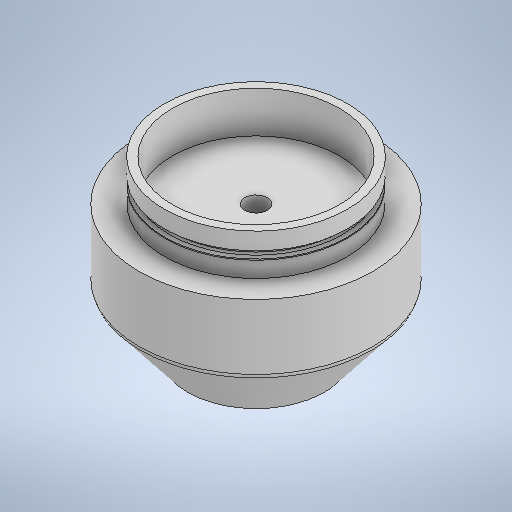
# Autodesk Inventor part: cap_v0.7.0
Saved by Autodesk Inventor 2025 (Build 290162000, 162)
## iProperties
Created: 2026-01-06
Part Number: cap_v0.7.0
Material: Generic
Document SubType Name: Modeling
Designer: SLM30
Density: 1 g/cm^3
Appearance: Default
Author: SLM30
Autodesk Inventor part; units mm, degrees
ref_plane "YZ Plane" through (0, 0, 0) normal (1, 0, 0) x (0, 1, 0)
ref_plane "XZ Plane" through (0, 0, 0) normal (0, 1, 0) x (-1, 0, 0)
ref_plane "XY Plane" through (0, 0, 0) normal (0, 0, 1) x (1, 0, 0)
sketch "Sketch1" plane through (0, 0, 0) normal (0, 0, 1) x (1, 0, 0)
  line L0 (0, 0) -> (-15, 0)
  line L1 (-15, 0) -> (-15, 11)
  line L2 (-15, 11) -> (-0.0863, 11)
  line L3 (-0.0863, 11) -> (-0.0863, 21)
  line L4 (-0.0863, 21) -> (-26.0863, 21)
  line L5 (-26.0863, 21) -> (-26.0863, 25.2964)
  line L6 (-26.0863, 25.2964) -> (-27.3219, 25.2964)
  line L7 (-28.5, 25.9476) -> (-28.5, 21)
  line L8 (-28.5, 21) -> (-36.5, 21)
  line L9 (-36.5, 21) -> (-36.5, 0)
  line L10 (-36.5, 0) -> (0, 0)
  line L11 (0, 0) -> (0, 0)
  line L12 (-36.5, 0) -> (-20.7775, -20)
  line L13 (-20.7775, -20) -> (0, -20)
  line L14 (0, -20) -> (0, 0)
  line L15 (-26.0863, 25.2964) -> (-26.0863, 33.8784)
  line L16 (-26.0863, 33.8784) -> (-28.5863, 33.8784)
  line L17 (-28.5863, 33.8784) -> (-28.5, 25.9476)
  arc A0 (-26.6145, 26.2707) -> (-28.5281, 28.5284) centre (-28.32, 26.765) ccw
  line L18 (-28.5, 24.9985) -> (-28.5035, 26.2655)
  line L19 (-28.5035, 26.2655) -> (-26.6145, 26.2707)
  line L20 (0, -30.7757) -> (0, 44.654) projected
  dimension "d0" = 21
  dimension "d1" = 8
  dimension "d2" = 2.5
  dimension "d3" = 4.9476
  dimension "d4" = 26
  dimension "d5" = 10
  dimension "d6" = 11
  dimension "d7" = 15
  dimension "d8" = 20
  dimension "d9" = 21.5
  dimension "d10" = 128.172
  dimension "d18" = 2.5
  dimension "d19" = 8.582
  dimension "d20" = 3.53
  dimension "d21" = 1.7756
  dimension "d22" = 1.2356
  dimension "d23" = 5.765
  dimension "d24" = 1.267
  constraints: 40 end point, 13 perpendicular, 6 point on line, 2 horizontal, 2 point on circle, 1 centre point, 1 vertical
  measures "d0" distance of L8.end L9.end
  measures "d1" distance of L7.end L8.end
  measures "d2" distance of L5.end L7.start
  measures "d3" distance of L7.start L7.end
  measures "d4" distance of L3.end L4.end
  measures "d5" distance of L2.end L3.end
  measures "d6" distance of L0.end L1.end
  measures "d7" distance of L0.start L0.end
  measures "d8" vertical distance of L9.end L12.end
  measures "d9" distance between parallel lines of L9 L1
  measures "d10" angle of L10 L12
  measures "d18" distance of L15.end L16.end
  measures "d19" distance of L5.end L15.end
  measures "d20" distance of L18.start A0.end
  measures "d21" radius of A0
  measures "d22" distance of L6.end L5.end
  measures "d23" distance from line of L8 A0.centre
  measures "d24" distance of L18.start L18.end
revolve "Revolution1" add sketch "Sketch1" angle 360 about axis through (0, -10, 0) along (0, 1, 0) contours L14 L13 L12 L10 L0 | L10 L9 L8 L7 L17 L19 A0 L16 L15 L5 L4 L3 L2 L1
fillet "Fillet1" radius 0.5 1 edges at (26.6145, 26.2707, 0)
fillet "Fillet2" radius 2 1 edges at (36.5, 0, 0)
fillet "Fillet3" radius 2 1 edges at (20.7775, -20, 0)
sketch "Sketch4" plane through (0, 21, 0) normal (0, 1, 0) x (1, 0, 0)
  circle A0 centre (0, 0) radius 3.5
  dimension "d28" = 7
  constraints: 1 centre point, 1 coincident
  measures "d28" diameter of A0
extrude "Extrusion3" cut sketch "Sketch4" against normal blind 10
sketch "Sketch5" plane through (0, -20, 0) normal (0, -1, 0) x (1, 0, 0)
  circle A0 centre (0, 0) radius 3.5 projected
  circle A1 centre (0, 0) radius 7
  dimension "d31" = 14
  constraints: 1 centre point, 1 coincident
  measures "d31" diameter of A1
extrude "Extrusion4" cut sketch "Sketch5" against normal blind 20 contours A0 | A1
body "Solid1"
